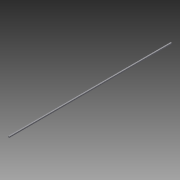
# Autodesk Inventor part: Part4
Saved by Autodesk Inventor 2014 (Build 180170000, 170)
## iProperties
Created: 2014-01-29
Part Number: Part4
Material: Generic
Document SubType Name: Modeling
Designer: NilesStanton
Density: 1 g/cm^3
Appearance: Default
Author: NilesStanton
Autodesk Inventor part; units mm, degrees
ref_plane "YZ Plane" through (0, 0, 0) normal (1, 0, 0) x (0, 1, 0)
ref_plane "XZ Plane" through (0, 0, 0) normal (0, 1, 0) x (-1, 0, 0)
ref_plane "XY Plane" through (0, 0, 0) normal (0, 0, 1) x (1, 0, 0)
sketch "Sketch1" plane through (0, 0, 0) normal (0, 1, 0) x (-1, 0, 0)
  line L0 (-326.5715, -322.2171) -> (-332.9215, -322.2171)
  line L1 (-332.9215, -322.2171) -> (-332.9215, 592.1829)
  line L2 (-332.9215, 592.1829) -> (-326.5715, 592.1829)
  line L3 (-326.5715, 592.1829) -> (-326.5715, -322.2171)
  point P0 (0, 0)
  dimension "d0" = 914.4
  dimension "d1" = 6.35
  constraints: 8 end point, 2 parallel, 1 horizontal, 1 perpendicular
  measures "d0" distance of L2.end L0.start
  measures "d1" distance of L0.start L0.end
extrude "Extrusion1" add sketch "Sketch1" along normal blind 6.35
body "Solid1"
